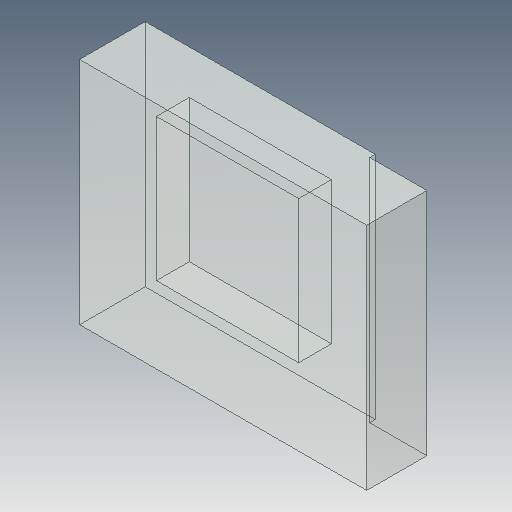
# Autodesk Inventor part: epoxy
Saved by Autodesk Inventor 2018.2 (Build 222227000, 227)
## iProperties
Created: 2016-03-28
Part Number: epoxy
Material: Glass
Document SubType Name: Modeling
Designer: sawai
Density: 2.18 g/cm^3
Appearance: Clear
Author: sawai
Autodesk Inventor part; units mm, degrees
ref_plane "YZ Plane" through (0, 0, 0) normal (1, 0, 0) x (0, 1, 0)
sketch "Sketch1" plane through (0, 0, 0) normal (0, 0, 1) x (1, 0, 0)
  line L0 (1.5725, 1.05) -> (1.05, 1.05) projected
  line L1 (1.05, 1.05) -> (1.05, -1.05) projected
  line L2 (1.05, -1.05) -> (1.5725, -1.05) projected
  line L3 (1.5725, -1.05) -> (1.5725, 1.05) projected
  line L4 (1.05, -1.05) -> (1.05, 1.05) projected
  line L5 (-1.0525, 1.05) -> (1.05, 1.05) projected
  line L6 (-1.0525, -1.05) -> (-1.0525, 1.05) projected
  line L7 (1.05, -1.05) -> (-1.0525, -1.05) projected
  line L8 (-0.65, -0.65) -> (0.65, -0.65) projected
  line L9 (-0.65, 0.65) -> (-0.65, -0.65) projected
  line L10 (0.65, 0.65) -> (-0.65, 0.65) projected
  line L11 (0.65, -0.65) -> (0.65, 0.65) projected
  point P0 (0, 0)
extrude "Extrusion1" add sketch "Sketch1" along normal blind 0.3 contours L3 L2 L1 L0 | L1 L7 L6 L5 | L9 L10 L11 L8
sketch "Sketch2" plane through (0, 0, 0) normal (0, 0, -1) x (-1, 0, 0)
  line L0 (-1.5725, 1.05) -> (-1.05, 1.05)
  line L1 (-1.05, 1.05) -> (-1.05, -1.05)
  line L2 (-1.05, -1.05) -> (-1.5725, -1.05)
  line L3 (-1.5725, -1.05) -> (-1.5725, 1.05)
  point P0 (0, 0)
  constraints: 8 end point
ref_plane "Work Plane1" through (1.05, -1.05, -0.25) normal (0, 0, 1) x (1, 0, 0)
extrude "Extrusion2" add sketch "Sketch2" along normal up to surface (0.25 mm away)
sketch "Sketch3" plane through (0, 0, 0) normal (0, 0, -1) x (-1, 0, 0)
  line L0 (-1.05, -1.05) -> (-1.05, 1.05)
  line L1 (1.0525, 1.05) -> (-1.05, 1.05)
  line L2 (1.0525, -1.05) -> (1.0525, 1.05)
  line L3 (-1.05, -1.05) -> (1.0525, -1.05)
  line L4 (0.65, -0.65) -> (-0.65, -0.65)
  line L5 (0.65, 0.65) -> (0.65, -0.65)
  line L6 (-0.65, 0.65) -> (0.65, 0.65)
  line L7 (-0.65, -0.65) -> (-0.65, 0.65)
  point P0 (0, 0)
  constraints: 16 end point
ref_plane "Work Plane2" through (-1.0525, -1.05, -0.3) normal (0, 0, 1) x (1, 0, 0)
extrude "Extrusion3" add sketch "Sketch3" along normal up to surface (0.3 mm away)
body "Solid1"
